Autodesk Fusion 360 part; units mm, degrees
(part 2 of 2)
  spline S177 degree 3 poles (-149.504, -22.8895) (-149.4923, -22.9168) (-149.4677, -22.974) (-149.4591, -23.0358) (-149.4546, -23.0681) knots 0 0 0 0 0.008862 0.018609 0.018609 0.018609 0.018609
  spline S178 degree 3 poles (-149.4546, -23.0681) (-149.4113, -23.0329) (-149.3307, -22.9673) (-149.2361, -22.924) (-149.1923, -22.9039) knots 0 0 0 0 0.016644 0.031058 0.031058 0.031058 0.031058
  spline S179 degree 3 poles (-149.1923, -22.9039) (-149.149, -22.8899) (-149.061, -22.8614) (-148.9686, -22.8576) (-148.9215, -22.8557) knots 0 0 0 0 0.013561 0.027613 0.027613 0.027613 0.027613
  spline S180 degree 3 poles (-148.9215, -22.8557) (-148.8489, -22.8584) (-148.7153, -22.8635) (-148.6047, -22.9378) (-148.5543, -22.9716) knots 0 0 0 0 0.021312 0.039186 0.039186 0.039186 0.039186
  spline S181 degree 3 poles (-148.5543, -22.9716) (-148.5169, -23.0135) (-148.4409, -23.0984) (-148.4307, -23.212) (-148.4255, -23.2695) knots 0 0 0 0 0.016401 0.033233 0.033233 0.033233 0.033233
  spline S182 degree 3 poles (-148.4255, -23.2695) (-148.4274, -23.3039) (-148.431, -23.3719) (-148.4595, -23.4336) (-148.4736, -23.464) knots 0 0 0 0 0.010253 0.020199 0.020199 0.020199 0.020199
  spline S183 degree 3 poles (-148.4736, -23.464) (-148.4907, -23.4917) (-148.5245, -23.5465) (-148.5752, -23.586) (-148.6002, -23.6054) knots 0 0 0 0 0.009704 0.019119 0.019119 0.019119 0.019119
  spline S184 degree 3 poles (-148.6002, -23.6054) (-148.6274, -23.6222) (-148.6829, -23.6564) (-148.7451, -23.6762) (-148.7767, -23.6862) knots 0 0 0 0 0.009559 0.019479 0.019479 0.019479 0.019479
  spline S185 degree 3 poles (-148.7767, -23.6862) (-148.8069, -23.6929) (-148.879, -23.709) (-148.9523, -23.7182) (-148.9949, -23.7235) knots 0 0 0 0 0.009264 0.022147 0.022147 0.022147 0.022147
  spline S186 degree 3 poles (-148.9949, -23.7235) (-149.0815, -23.7341) (-149.2295, -23.7523) (-149.3731, -23.7923) (-149.4327, -23.8089) knots 0 0 0 0 0.02611 0.044656 0.044656 0.044656 0.044656
  spline S187 degree 3 poles (-149.4327, -23.8089) (-149.4331, -23.8227) (-149.4336, -23.844) (-149.4338, -23.8654) (-149.4339, -23.873) knots 0 0 0 0 0.004128 0.006413 0.006413 0.006413 0.006413
  spline S188 degree 3 poles (-149.4339, -23.873) (-149.4329, -23.9174) (-149.431, -23.9956) (-149.3842, -24.0575) (-149.364, -24.0843) knots 0 0 0 0 0.012908 0.022759 0.022759 0.022759 0.022759
  spline S189 degree 3 poles (-149.364, -24.0843) (-149.326, -24.1085) (-149.2411, -24.1625) (-149.14, -24.1654) (-149.0841, -24.167) knots 0 0 0 0 0.013259 0.029661 0.029661 0.029661 0.029661
  spline S190 degree 3 poles (-149.0841, -24.167) (-149.0328, -24.1661) (-148.9427, -24.1646) (-148.8628, -24.1235) (-148.8284, -24.1058) knots 0 0 0 0 0.015134 0.026599 0.026599 0.026599 0.026599
  spline S191 degree 3 poles (-148.8284, -24.1058) (-148.8022, -24.0792) (-148.7427, -24.0187) (-148.7196, -23.9366) (-148.7068, -23.8907) knots 0 0 0 0 0.011056 0.025069 0.025069 0.025069 0.025069
  line L112 (-148.7068, -23.8907) -> (-148.4666, -23.923)
  spline S192 degree 3 poles (-148.4666, -23.923) (-148.4782, -23.9707) (-148.5, -24.0599) (-148.5504, -24.1365) (-148.5739, -24.1722) knots 0 0 0 0 0.01459 0.02731 0.02731 0.02731 0.02731
  spline S193 degree 3 poles (-148.5739, -24.1722) (-148.6029, -24.2025) (-148.6644, -24.2668) (-148.7469, -24.3007) (-148.7905, -24.3186) knots 0 0 0 0 0.012433 0.026404 0.026404 0.026404 0.026404
  spline S194 degree 3 poles (-148.7905, -24.3186) (-148.8412, -24.3336) (-148.9484, -24.3653) (-149.0602, -24.3686) (-149.1192, -24.3704) knots 0 0 0 0 0.015787 0.033398 0.033398 0.033398 0.033398
  spline S195 degree 3 poles (-149.1192, -24.3704) (-149.1757, -24.3695) (-149.2782, -24.368) (-149.3766, -24.3399) (-149.4208, -24.3273) knots 0 0 0 0 0.01685 0.030582 0.030582 0.030582 0.030582
  spline S196 degree 3 poles (-149.4208, -24.3273) (-149.4558, -24.3131) (-149.5197, -24.2873) (-149.5692, -24.2394) (-149.5915, -24.2178) knots 0 0 0 0 0.011204 0.020452 0.020452 0.020452 0.020452
  spline S197 degree 3 poles (-149.5915, -24.2178) (-149.6086, -24.1936) (-149.6443, -24.1427) (-149.66, -24.0824) (-149.6682, -24.0508) knots 0 0 0 0 0.008807 0.018509 0.018509 0.018509 0.018509
  spline S198 degree 3 poles (-149.6682, -24.0508) (-149.6718, -24.0215) (-149.6811, -23.9464) (-149.681, -23.8706) (-149.681, -23.8244) knots 0 0 0 0 0.008847 0.022698 0.022698 0.022698 0.022698
  line L113 (-149.681, -23.8244) -> (-149.6816, -23.497)
  spline S199 degree 3 poles (-149.6816, -23.497) (-149.6812, -23.4037) (-149.6806, -23.259) (-149.6935, -23.115) (-149.6981, -23.0638) knots 0 0 0 0 0.027953 0.043363 0.043363 0.043363 0.043363
  spline S200 degree 3 poles (-149.6981, -23.0638) (-149.7047, -23.0338) (-149.7181, -22.9732) (-149.7463, -22.9179) (-149.7605, -22.89) knots 0 0 0 0 0.009187 0.018535 0.018535 0.018535 0.018535
  spline S201 degree 3 poles (-144.8078, -22.2926) (-144.7279, -22.2957) (-144.5787, -22.3016) (-144.449, -22.3746) (-144.3888, -22.4085) knots 0 0 0 0 0.023612 0.044032 0.044032 0.044032 0.044032
  spline S202 degree 3 poles (-144.3888, -22.4085) (-144.3425, -22.454) (-144.2448, -22.55) (-144.2377, -22.6873) (-144.234, -22.7595) knots 0 0 0 0 0.018806 0.039631 0.039631 0.039631 0.039631
  line L114 (-144.234, -22.7595) -> (-144.4728, -22.7244)
  spline S203 degree 3 poles (-144.4728, -22.7244) (-144.4791, -22.6909) (-144.4908, -22.6286) (-144.5356, -22.5841) (-144.5563, -22.5636) knots 0 0 0 0 0.009961 0.018507 0.018507 0.018507 0.018507
  spline S204 degree 3 poles (-144.5563, -22.5636) (-144.5916, -22.5438) (-144.6689, -22.5005) (-144.7578, -22.4975) (-144.8061, -22.4959) knots 0 0 0 0 0.011961 0.026218 0.026218 0.026218 0.026218
  spline S205 degree 3 poles (-144.8061, -22.4959) (-144.8576, -22.4974) (-144.951, -22.5002) (-145.0327, -22.5447) (-145.0693, -22.5646) knots 0 0 0 0 0.015205 0.027537 0.027537 0.027537 0.027537
  spline S206 degree 3 poles (-145.0693, -22.5646) (-145.0978, -22.5902) (-145.1564, -22.6428) (-145.1815, -22.7175) (-145.1944, -22.7558) knots 0 0 0 0 0.01129 0.023203 0.023203 0.023203 0.023203
  spline S207 degree 3 poles (-145.1944, -22.7558) (-145.1997, -22.7946) (-145.2141, -22.899) (-145.2125, -23.0046) (-145.2115, -23.071) knots 0 0 0 0 0.011714 0.031602 0.031602 0.031602 0.031602
  spline S208 degree 3 poles (-145.2115, -23.071) (-145.1551, -23.0156) (-145.0434, -22.9059) (-144.8878, -22.889) (-144.8108, -22.8806) knots 0 0 0 0 0.023001 0.045538 0.045538 0.045538 0.045538
  spline S209 degree 3 poles (-144.8108, -22.8806) (-144.7177, -22.8883) (-144.5367, -22.9033) (-144.4096, -23.0325) (-144.3479, -23.0953) knots 0 0 0 0 0.027043 0.052564 0.052564 0.052564 0.052564
  spline S210 degree 3 poles (-144.3479, -23.0953) (-144.3, -23.172) (-144.2014, -23.3301) (-144.1894, -23.5162) (-144.1832, -23.612) knots 0 0 0 0 0.026695 0.054994 0.054994 0.054994 0.054994
  spline S211 degree 3 poles (-144.1832, -23.612) (-144.186, -23.6792) (-144.1913, -23.8106) (-144.2358, -23.9343) (-144.2575, -23.9948) knots 0 0 0 0 0.020023 0.0392 0.0392 0.0392 0.0392
  spline S212 degree 3 poles (-144.2575, -23.9948) (-144.2846, -24.0495) (-144.3371, -24.1559) (-144.4297, -24.23) (-144.4746, -24.2661) knots 0 0 0 0 0.018051 0.035117 0.035117 0.035117 0.035117
  spline S213 degree 3 poles (-144.4746, -24.2661) (-144.5251, -24.294) (-144.6292, -24.3516) (-144.7481, -24.3586) (-144.8094, -24.3622) knots 0 0 0 0 0.017076 0.035225 0.035225 0.035225 0.035225
  spline S214 degree 3 poles (-144.8094, -24.3622) (-144.8914, -24.3534) (-145.0572, -24.3355) (-145.1738, -24.216) (-145.2327, -24.1556) knots 0 0 0 0 0.023964 0.048437 0.048437 0.048437 0.048437
  line L115 (-145.2327, -24.1556) -> (-145.2323, -24.3303)
  line L116 (-145.2323, -24.3303) -> (-145.4588, -24.3307)
  line L117 (-145.4588, -24.3307) -> (-145.4612, -23.0783)
  spline S215 degree 3 poles (-145.4612, -23.0783) (-145.4614, -22.981) (-145.4619, -22.8174) (-145.413, -22.6617) (-145.3932, -22.5986) knots 0 0 0 0 0.028956 0.048693 0.048693 0.048693 0.048693
  spline S216 degree 3 poles (-145.3932, -22.5986) (-145.3665, -22.5537) (-145.3118, -22.4619) (-145.2215, -22.4045) (-145.1754, -22.3752) knots 0 0 0 0 0.015457 0.0316 0.0316 0.0316 0.0316
  spline S217 degree 3 poles (-145.1754, -22.3752) (-145.1206, -22.3512) (-145.0037, -22.3) (-144.8759, -22.2952) (-144.8078, -22.2926) knots 0 0 0 0 0.017756 0.037966 0.037966 0.037966 0.037966
  line L118 (-143.0208, -22.8772) -> (-142.7643, -22.8767)
  spline S218 degree 3 poles (-142.7643, -22.8767) (-142.7526, -22.904) (-142.728, -22.9612) (-142.7194, -23.023) (-142.7149, -23.0554) knots 0 0 0 0 0.008862 0.018609 0.018609 0.018609 0.018609
  spline S219 degree 3 poles (-142.7149, -23.0554) (-142.6716, -23.0201) (-142.591, -22.9545) (-142.4964, -22.9112) (-142.4526, -22.8911) knots 0 0 0 0 0.016644 0.031058 0.031058 0.031058 0.031058
  spline S220 degree 3 poles (-142.4526, -22.8911) (-142.4093, -22.8771) (-142.3213, -22.8486) (-142.2289, -22.8448) (-142.1819, -22.8429) knots 0 0 0 0 0.013561 0.027613 0.027613 0.027613 0.027613
  spline S221 degree 3 poles (-142.1819, -22.8429) (-142.1092, -22.8456) (-141.9756, -22.8507) (-141.8651, -22.925) (-141.8146, -22.9588) knots 0 0 0 0 0.021312 0.039186 0.039186 0.039186 0.039186
  spline S222 degree 3 poles (-141.8146, -22.9588) (-141.7772, -23.0007) (-141.7012, -23.0856) (-141.691, -23.1992) (-141.6858, -23.2567) knots 0 0 0 0 0.016401 0.033233 0.033233 0.033233 0.033233
  spline S223 degree 3 poles (-141.6858, -23.2567) (-141.6877, -23.2911) (-141.6913, -23.3591) (-141.7198, -23.4208) (-141.7339, -23.4512) knots 0 0 0 0 0.010253 0.020199 0.020199 0.020199 0.020199
  spline S224 degree 3 poles (-141.7339, -23.4512) (-141.751, -23.4789) (-141.7848, -23.5337) (-141.8355, -23.5732) (-141.8605, -23.5926) knots 0 0 0 0 0.009704 0.019119 0.019119 0.019119 0.019119
  spline S225 degree 3 poles (-141.8605, -23.5926) (-141.8877, -23.6094) (-141.9432, -23.6436) (-142.0054, -23.6634) (-142.037, -23.6734) knots 0 0 0 0 0.009559 0.019479 0.019479 0.019479 0.019479
  spline S226 degree 3 poles (-142.037, -23.6734) (-142.0672, -23.6801) (-142.1393, -23.6962) (-142.2126, -23.7054) (-142.2552, -23.7107) knots 0 0 0 0 0.009264 0.022147 0.022147 0.022147 0.022147
  spline S227 degree 3 poles (-142.2552, -23.7107) (-142.3418, -23.7213) (-142.4898, -23.7395) (-142.6334, -23.7795) (-142.693, -23.7961) knots 0 0 0 0 0.02611 0.044656 0.044656 0.044656 0.044656
  spline S228 degree 3 poles (-142.693, -23.7961) (-142.6934, -23.8099) (-142.6939, -23.8312) (-142.6942, -23.8526) (-142.6942, -23.8602) knots 0 0 0 0 0.004128 0.006413 0.006413 0.006413 0.006413
  spline S229 degree 3 poles (-142.6942, -23.8602) (-142.6932, -23.9046) (-142.6913, -23.9828) (-142.6445, -24.0448) (-142.6243, -24.0716) knots 0 0 0 0 0.012908 0.022759 0.022759 0.022759 0.022759
  spline S230 degree 3 poles (-142.6243, -24.0716) (-142.5863, -24.0957) (-142.5014, -24.1497) (-142.4003, -24.1526) (-142.3444, -24.1542) knots 0 0 0 0 0.013259 0.029661 0.029661 0.029661 0.029661
  spline S231 degree 3 poles (-142.3444, -24.1542) (-142.2931, -24.1533) (-142.203, -24.1518) (-142.1232, -24.1107) (-142.0888, -24.093) knots 0 0 0 0 0.015134 0.026599 0.026599 0.026599 0.026599
  spline S232 degree 3 poles (-142.0888, -24.093) (-142.0625, -24.0664) (-142.003, -24.0059) (-141.98, -23.9238) (-141.9671, -23.8779) knots 0 0 0 0 0.011056 0.025069 0.025069 0.025069 0.025069
  line L119 (-141.9671, -23.8779) -> (-141.7269, -23.9102)
  spline S233 degree 3 poles (-141.7269, -23.9102) (-141.7385, -23.9579) (-141.7603, -24.0471) (-141.8107, -24.1237) (-141.8342, -24.1594) knots 0 0 0 0 0.01459 0.02731 0.02731 0.02731 0.02731
  spline S234 degree 3 poles (-141.8342, -24.1594) (-141.8632, -24.1897) (-141.9247, -24.254) (-142.0072, -24.2879) (-142.0508, -24.3058) knots 0 0 0 0 0.012433 0.026404 0.026404 0.026404 0.026404
  spline S235 degree 3 poles (-142.0508, -24.3058) (-142.1015, -24.3208) (-142.2087, -24.3525) (-142.3206, -24.3558) (-142.3795, -24.3576) knots 0 0 0 0 0.015787 0.033398 0.033398 0.033398 0.033398
  spline S236 degree 3 poles (-142.3795, -24.3576) (-142.436, -24.3567) (-142.5385, -24.3552) (-142.6369, -24.3271) (-142.6811, -24.3145) knots 0 0 0 0 0.01685 0.030582 0.030582 0.030582 0.030582
  spline S237 degree 3 poles (-142.6811, -24.3145) (-142.7161, -24.3003) (-142.78, -24.2745) (-142.8295, -24.2266) (-142.8518, -24.205) knots 0 0 0 0 0.011204 0.020452 0.020452 0.020452 0.020452
  spline S238 degree 3 poles (-142.8518, -24.205) (-142.8689, -24.1808) (-142.9047, -24.1299) (-142.9203, -24.0696) (-142.9286, -24.038) knots 0 0 0 0 0.008807 0.018509 0.018509 0.018509 0.018509
  spline S239 degree 3 poles (-142.9286, -24.038) (-142.9322, -24.0087) (-142.9414, -23.9336) (-142.9413, -23.8578) (-142.9413, -23.8116) knots 0 0 0 0 0.008847 0.022698 0.022698 0.022698 0.022698
  line L120 (-142.9413, -23.8116) -> (-142.9419, -23.4842)
  spline S240 degree 3 poles (-142.9419, -23.4842) (-142.9415, -23.3909) (-142.9409, -23.2462) (-142.9538, -23.1022) (-142.9584, -23.051) knots 0 0 0 0 0.027953 0.043363 0.043363 0.043363 0.043363
  spline S241 degree 3 poles (-142.9584, -23.051) (-142.965, -23.021) (-142.9784, -22.9604) (-143.0066, -22.9051) (-143.0208, -22.8772) knots 0 0 0 0 0.009187 0.018535 0.018535 0.018535 0.018535
  spline S242 degree 3 poles (-148.8692, -25.9756) (-148.7958, -25.9798) (-148.6557, -25.9878) (-148.5405, -26.0673) (-148.4856, -26.1052) knots 0 0 0 0 0.021564 0.041189 0.041189 0.041189 0.041189
  spline S243 degree 3 poles (-148.4856, -26.1052) (-148.4407, -26.1548) (-148.346, -26.2593) (-148.3199, -26.3982) (-148.3062, -26.4712) knots 0 0 0 0 0.01968 0.041471 0.041471 0.041471 0.041471
  line L121 (-148.3062, -26.4712) -> (-148.5421, -26.4934)
  spline S244 degree 3 poles (-148.5421, -26.4934) (-148.5527, -26.4436) (-148.5717, -26.3535) (-148.6308, -26.2834) (-148.6572, -26.2522) knots 0 0 0 0 0.015008 0.027097 0.027097 0.027097 0.027097
  spline S245 degree 3 poles (-148.6572, -26.2522) (-148.6883, -26.2304) (-148.7533, -26.1848) (-148.8328, -26.18) (-148.8743, -26.1776) knots 0 0 0 0 0.011173 0.023358 0.023358 0.023358 0.023358
  spline S246 degree 3 poles (-148.8743, -26.1776) (-148.9103, -26.1795) (-148.9801, -26.1832) (-149.0425, -26.2146) (-149.0727, -26.2298) knots 0 0 0 0 0.010703 0.020715 0.020715 0.020715 0.020715
  spline S247 degree 3 poles (-149.0727, -26.2298) (-149.0998, -26.2487) (-149.1545, -26.2867) (-149.1929, -26.3411) (-149.2122, -26.3685) knots 0 0 0 0 0.009841 0.019815 0.019815 0.019815 0.019815
  spline S248 degree 3 poles (-149.2122, -26.3685) (-149.2301, -26.402) (-149.2698, -26.4763) (-149.2913, -26.5579) (-149.3032, -26.6027) knots 0 0 0 0 0.011348 0.025194 0.025194 0.025194 0.025194
  spline S249 degree 3 poles (-149.3032, -26.6027) (-149.3138, -26.6521) (-149.3352, -26.751) (-149.338, -26.8522) (-149.3394, -26.9029) knots 0 0 0 0 0.015125 0.030296 0.030296 0.030296 0.030296
  spline S250 degree 3 poles (-149.3394, -26.9029) (-149.3394, -26.9097) (-149.3391, -26.9261) (-149.3384, -26.9424) (-149.338, -26.952) knots 0 0 0 0 0.002047 0.004913 0.004913 0.004913 0.004913
  spline S251 degree 3 poles (-149.338, -26.952) (-149.3109, -26.9145) (-149.256, -26.8383) (-149.1772, -26.7872) (-149.1371, -26.7613) knots 0 0 0 0 0.013741 0.027912 0.027912 0.027912 0.027912
  spline S252 degree 3 poles (-149.1371, -26.7613) (-149.0937, -26.7399) (-149.0065, -26.697) (-148.9096, -26.6909) (-148.861, -26.6878) knots 0 0 0 0 0.014368 0.028825 0.028825 0.028825 0.028825
  spline S253 degree 3 poles (-148.861, -26.6878) (-148.7814, -26.6951) (-148.622, -26.7099) (-148.501, -26.8146) (-148.4405, -26.867) knots 0 0 0 0 0.023358 0.04675 0.04675 0.04675 0.04675
  spline S254 degree 3 poles (-148.4405, -26.867) (-148.3902, -26.9339) (-148.2848, -27.0741) (-148.2736, -27.2496) (-148.2677, -27.3415) knots 0 0 0 0 0.024534 0.051481 0.051481 0.051481 0.051481
  spline S255 degree 3 poles (-148.2677, -27.3415) (-148.2735, -27.4364) (-148.2846, -27.6179) (-148.394, -27.7626) (-148.4461, -27.8316) knots 0 0 0 0 0.02782 0.053201 0.053201 0.053201 0.053201
  spline S256 degree 3 poles (-148.4461, -27.8316) (-148.5102, -27.8858) (-148.6399, -27.9957) (-148.8095, -28.0105) (-148.8953, -28.018) knots 0 0 0 0 0.024536 0.049711 0.049711 0.049711 0.049711
  spline S257 degree 3 poles (-148.8953, -28.018) (-148.9589, -28.0138) (-149.0856, -28.0054) (-149.1968, -27.9441) (-149.2523, -27.9136) knots 0 0 0 0 0.018857 0.037596 0.037596 0.037596 0.037596
  spline S258 degree 3 poles (-149.2523, -27.9136) (-149.3033, -27.8742) (-149.408, -27.7933) (-149.4678, -27.6752) (-149.4984, -27.6146) knots 0 0 0 0 0.019093 0.039165 0.039165 0.039165 0.039165
  spline S259 degree 3 poles (-149.4984, -27.6146) (-149.5229, -27.5359) (-149.5798, -27.3531) (-149.5821, -27.1613) (-149.5834, -27.052) knots 0 0 0 0 0.024607 0.057161 0.057161 0.057161 0.057161
  spline S260 degree 3 poles (-149.5834, -27.052) (-149.582, -26.9365) (-149.5797, -26.7293) (-149.5253, -26.5297) (-149.5013, -26.4414) knots 0 0 0 0 0.034493 0.061835 0.061835 0.061835 0.061835
  spline S261 degree 3 poles (-149.5013, -26.4414) (-149.4717, -26.3712) (-149.4152, -26.237) (-149.3063, -26.1409) (-149.2544, -26.0951) knots 0 0 0 0 0.022523 0.043023 0.043023 0.043023 0.043023
  spline S262 degree 3 poles (-149.2544, -26.0951) (-149.1964, -26.0603) (-149.0779, -25.9892) (-148.9398, -25.9802) (-148.8692, -25.9756) knots 0 0 0 0 0.019951 0.040848 0.040848 0.040848 0.040848
  spline S263 degree 3 poles (-146.7002, -26.5841) (-146.7034, -26.6454) (-146.7095, -26.7626) (-146.7697, -26.863) (-146.7984, -26.911) knots 0 0 0 0 0.018093 0.034604 0.034604 0.034604 0.034604
  spline S264 degree 3 poles (-146.7984, -26.911) (-146.8359, -26.9517) (-146.9137, -27.0363) (-147.0231, -27.0723) (-147.0798, -27.0909) knots 0 0 0 0 0.016316 0.033898 0.033898 0.033898 0.033898
  spline S265 degree 3 poles (-147.0798, -27.0909) (-147.0331, -27.1102) (-146.9454, -27.1464) (-146.8825, -27.2171) (-146.8531, -27.2501) knots 0 0 0 0 0.014933 0.028029 0.028029 0.028029 0.028029
  spline S266 degree 3 poles (-146.8531, -27.2501) (-146.8315, -27.2871) (-146.7869, -27.3638) (-146.7816, -27.4524) (-146.7789, -27.4983) knots 0 0 0 0 0.012661 0.026224 0.026224 0.026224 0.026224
  spline S267 degree 3 poles (-146.7789, -27.4983) (-146.7852, -27.5681) (-146.7979, -27.7073) (-146.8894, -27.8129) (-146.9351, -27.8656) knots 0 0 0 0 0.020468 0.040823 0.040823 0.040823 0.040823
  spline S268 degree 3 poles (-146.9351, -27.8656) (-146.9937, -27.909) (-147.1173, -28.0007) (-147.2713, -28.0101) (-147.3523, -28.0151) knots 0 0 0 0 0.021415 0.045172 0.045172 0.045172 0.045172
  spline S269 degree 3 poles (-147.3523, -28.0151) (-147.4339, -28.0102) (-147.5897, -28.0009) (-147.7147, -27.908) (-147.7741, -27.8637) knots 0 0 0 0 0.02394 0.045691 0.045691 0.045691 0.045691
  spline S270 degree 3 poles (-147.7741, -27.8637) (-147.8208, -27.8105) (-147.9138, -27.7042) (-147.9276, -27.5637) (-147.9345, -27.4936) knots 0 0 0 0 0.020682 0.041247 0.041247 0.041247 0.041247
  spline S271 degree 3 poles (-147.9345, -27.4936) (-147.9318, -27.4492) (-147.9267, -27.3627) (-147.8831, -27.2878) (-147.8619, -27.2514) knots 0 0 0 0 0.013139 0.025609 0.025609 0.025609 0.025609
  spline S272 degree 3 poles (-147.8619, -27.2514) (-147.8331, -27.2184) (-147.7718, -27.1483) (-147.686, -27.1115) (-147.6405, -27.092) knots 0 0 0 0 0.012951 0.027588 0.027588 0.027588 0.027588
  spline S273 degree 3 poles (-147.6405, -27.092) (-147.6975, -27.0701) (-147.8067, -27.0281) (-147.8842, -26.9406) (-147.9213, -26.8988) knots 0 0 0 0 0.018015 0.034524 0.034524 0.034524 0.034524
  spline S274 degree 3 poles (-147.9213, -26.8988) (-147.9494, -26.8512) (-148.0075, -26.7528) (-148.0145, -26.6387) (-148.018, -26.5798) knots 0 0 0 0 0.016344 0.033768 0.033768 0.033768 0.033768
  spline S275 degree 3 poles (-148.018, -26.5798) (-148.0108, -26.4978) (-147.9964, -26.3348) (-147.8902, -26.2102) (-147.8374, -26.1483) knots 0 0 0 0 0.024034 0.04782 0.04782 0.04782 0.04782
  spline S276 degree 3 poles (-147.8374, -26.1483) (-147.7702, -26.0973) (-147.6294, -25.9904) (-147.4526, -25.9788) (-147.3603, -25.9728) knots 0 0 0 0 0.024757 0.051851 0.051851 0.051851 0.051851
  spline S277 degree 3 poles (-147.3603, -25.9728) (-147.2678, -25.9785) (-147.0909, -25.9895) (-146.9498, -26.0962) (-146.8824, -26.1472) knots 0 0 0 0 0.027096 0.051881 0.051881 0.051881 0.051881
  spline S278 degree 3 poles (-146.8824, -26.1472) (-146.8294, -26.2096) (-146.7222, -26.3357) (-146.7076, -26.5007) (-146.7002, -26.5841) knots 0 0 0 0 0.02394 0.048393 0.048393 0.048393 0.048393
  spline S279 degree 3 poles (-144.2237, -25.9668) (-144.1332, -25.9744) (-143.9567, -25.9891) (-143.8305, -26.113) (-143.769, -26.1733) knots 0 0 0 0 0.026334 0.051363 0.051363 0.051363 0.051363
  spline S280 degree 3 poles (-143.769, -26.1733) (-143.7115, -26.2804) (-143.5759, -26.5326) (-143.572, -26.8205) (-143.5697, -26.986) knots 0 0 0 0 0.036009 0.08476 0.08476 0.08476 0.08476
  spline S281 degree 3 poles (-143.5697, -26.986) (-143.5709, -27.0934) (-143.5732, -27.2867) (-143.6205, -27.4739) (-143.6416, -27.5571) knots 0 0 0 0 0.032061 0.057736 0.057736 0.057736 0.057736
  spline S282 degree 3 poles (-143.6416, -27.5571) (-143.6673, -27.6239) (-143.7161, -27.7506) (-143.8124, -27.846) (-143.8579, -27.8911) knots 0 0 0 0 0.021191 0.040192 0.040192 0.040192 0.040192
  spline S283 degree 3 poles (-143.8579, -27.8911) (-143.9104, -27.9254) (-144.0202, -27.9972) (-144.1514, -28.005) (-144.2199, -28.0091) knots 0 0 0 0 0.018481 0.038665 0.038665 0.038665 0.038665
  spline S284 degree 3 poles (-144.2199, -28.0091) (-144.271, -28.007) (-144.3692, -28.0029) (-144.4592, -27.9636) (-144.5024, -27.9448) knots 0 0 0 0 0.015196 0.029197 0.029197 0.029197 0.029197
  spline S285 degree 3 poles (-144.5024, -27.9448) (-144.5413, -27.9206) (-144.6204, -27.8715) (-144.6754, -27.7964) (-144.7033, -27.7583) knots 0 0 0 0 0.013619 0.027641 0.027641 0.027641 0.027641
  spline S286 degree 3 poles (-144.7033, -27.7583) (-144.7287, -27.714) (-144.7825, -27.6201) (-144.8123, -27.5161) (-144.828, -27.4611) knots 0 0 0 0 0.01527 0.032333 0.032333 0.032333 0.032333
  spline S287 degree 3 poles (-144.828, -27.4611) (-144.8412, -27.3927) (-144.8713, -27.2368) (-144.873, -27.0778) (-144.8739, -26.9885) knots 0 0 0 0 0.020858 0.04757 0.04757 0.04757 0.04757
  spline S288 degree 3 poles (-144.8739, -26.9885) (-144.8726, -26.8819) (-144.8704, -26.6896) (-144.8235, -26.5032) (-144.8027, -26.4202) knots 0 0 0 0 0.031856 0.057454 0.057454 0.057454 0.057454
  spline S289 degree 3 poles (-144.8027, -26.4202) (-144.7771, -26.3533) (-144.7286, -26.2265) (-144.6325, -26.1308) (-144.5871, -26.0855) knots 0 0 0 0 0.021185 0.040213 0.040213 0.040213 0.040213
  spline S290 degree 3 poles (-144.5871, -26.0855) (-144.5345, -26.051) (-144.4243, -25.9788) (-144.2926, -25.9709) (-144.2237, -25.9668) knots 0 0 0 0 0.018535 0.038823 0.038823 0.038823 0.038823
  spline S291 degree 3 poles (-140.9528, -26.3317) (-140.9886, -26.3949) (-141.0772, -26.5513) (-141.0764, -26.7327) (-141.076, -26.8408) knots 0 0 0 0 0.021463 0.053164 0.053164 0.053164 0.053164
  line L122 (-141.076, -26.8408) -> (-141.0738, -27.9949)
  line L123 (-141.0738, -27.9949) -> (-141.3385, -27.9954)
  line L124 (-141.3385, -27.9954) -> (-141.3406, -26.8399)
  spline S292 degree 3 poles (-141.3406, -26.8399) (-141.3396, -26.7491) (-141.3376, -26.5863) (-141.293, -26.43) (-141.2733, -26.3609) knots 0 0 0 0 0.0271 0.048558 0.048558 0.048558 0.048558
  spline S293 degree 3 poles (-141.2733, -26.3609) (-141.2454, -26.3041) (-141.1879, -26.1872) (-141.082, -26.111) (-141.0276, -26.0719) knots 0 0 0 0 0.018712 0.038457 0.038457 0.038457 0.038457
  spline S294 degree 3 poles (-141.0276, -26.0719) (-140.9602, -26.0394) (-140.813, -25.9685) (-140.6493, -25.9629) (-140.5606, -25.9599) knots 0 0 0 0 0.022208 0.048498 0.048498 0.048498 0.048498
  spline S295 degree 3 poles (-140.5606, -25.9599) (-140.4742, -25.9622) (-140.3148, -25.9665) (-140.1679, -26.0278) (-140.1007, -26.0558) knots 0 0 0 0 0.02566 0.047343 0.047343 0.047343 0.047343
  spline S296 degree 3 poles (-140.1007, -26.0558) (-140.0454, -26.0915) (-139.9354, -26.1622) (-139.875, -26.2781) (-139.845, -26.3357) knots 0 0 0 0 0.019364 0.038493 0.038493 0.038493 0.038493
  spline S297 degree 3 poles (-139.845, -26.3357) (-139.8227, -26.4075) (-139.772, -26.5705) (-139.7692, -26.7414) (-139.7677, -26.8369) knots 0 0 0 0 0.022452 0.050944 0.050944 0.050944 0.050944
  line L125 (-139.7677, -26.8369) -> (-139.7655, -27.9925)
  line L126 (-139.7655, -27.9925) -> (-140.0301, -27.993)
  line L127 (-140.0301, -27.993) -> (-140.0323, -26.8388)
  spline S298 degree 3 poles (-140.0323, -26.8388) (-140.0327, -26.7628) (-140.0334, -26.6326) (-140.0674, -26.5071) (-140.0815, -26.4549) knots 0 0 0 0 0.022662 0.038849 0.038849 0.038849 0.038849
  spline S299 degree 3 poles (-140.0815, -26.4549) (-140.1007, -26.416) (-140.1394, -26.3379) (-140.2119, -26.2893) (-140.2483, -26.2649) knots 0 0 0 0 0.01276 0.025677 0.025677 0.025677 0.025677
  spline S300 degree 3 poles (-140.2483, -26.2649) (-140.2914, -26.2455) (-140.383, -26.2042) (-140.4836, -26.2005) (-140.537, -26.1986) knots 0 0 0 0 0.01404 0.029868 0.029868 0.029868 0.029868
  spline S301 degree 3 poles (-140.537, -26.1986) (-140.6234, -26.2007) (-140.7763, -26.2044) (-140.8994, -26.2932) (-140.9528, -26.3317) knots 0 0 0 0 0.025218 0.044567 0.044567 0.044567 0.044567
  spline S302 degree 3 poles (-153.5723, -29.3325) (-153.6428, -29.3373) (-153.78, -29.3467) (-153.8935, -29.4239) (-153.9486, -29.4614) knots 0 0 0 0 0.020781 0.040419 0.040419 0.040419 0.040419
  spline S303 degree 3 poles (-153.9486, -29.4614) (-153.9963, -29.512) (-154.0985, -29.6205) (-154.1364, -29.7652) (-154.1566, -29.8424) knots 0 0 0 0 0.020513 0.044031 0.044031 0.044031 0.044031
  line L128 (-154.1566, -29.8424) -> (-154.4214, -29.7761)
  spline S304 degree 3 poles (-154.4214, -29.7761) (-154.3905, -29.6755) (-154.3317, -29.4847) (-154.19, -29.3446) (-154.1229, -29.2783) knots 0 0 0 0 0.031005 0.058853 0.058853 0.058853 0.058853
  spline S305 degree 3 poles (-154.1229, -29.2783) (-154.0453, -29.2282) (-153.8845, -29.1245) (-153.6934, -29.1123) (-153.5946, -29.106) knots 0 0 0 0 0.027244 0.056397 0.056397 0.056397 0.056397
  spline S306 degree 3 poles (-153.5946, -29.106) (-153.4949, -29.1094) (-153.3099, -29.1157) (-153.1447, -29.1985) (-153.0684, -29.2367) knots 0 0 0 0 0.029499 0.054784 0.054784 0.054784 0.054784
  spline S307 degree 3 poles (-153.0684, -29.2367) (-153.0043, -29.2866) (-152.8721, -29.3895) (-152.7977, -29.5399) (-152.7594, -29.6174) knots 0 0 0 0 0.024039 0.049604 0.049604 0.049604 0.049604
  spline S308 degree 3 poles (-152.7594, -29.6174) (-152.7284, -29.7028) (-152.6655, -29.8759) (-152.657, -30.06) (-152.6526, -30.1534) knots 0 0 0 0 0.027074 0.054928 0.054928 0.054928 0.054928
  spline S309 degree 3 poles (-152.6526, -30.1534) (-152.6564, -30.2522) (-152.6637, -30.4411) (-152.7363, -30.6155) (-152.771, -30.6986) knots 0 0 0 0 0.029398 0.056194 0.056194 0.056194 0.056194
  spline S310 degree 3 poles (-152.771, -30.6986) (-152.8144, -30.7713) (-152.9004, -30.9153) (-153.0406, -31.0071) (-153.11, -31.0526) knots 0 0 0 0 0.025058 0.049588 0.049588 0.049588 0.049588
  spline S311 degree 3 poles (-153.11, -31.0526) (-153.1858, -31.0879) (-153.3395, -31.1596) (-153.5089, -31.1693) (-153.5948, -31.1742) knots 0 0 0 0 0.02485 0.050387 0.050387 0.050387 0.050387
  spline S312 degree 3 poles (-153.5948, -31.1742) (-153.6892, -31.1692) (-153.8702, -31.1597) (-154.0255, -31.0668) (-154.0998, -31.0224) knots 0 0 0 0 0.027889 0.053453 0.053453 0.053453 0.053453
  spline S313 degree 3 poles (-154.0998, -31.0224) (-154.1634, -30.965) (-154.2948, -30.8463) (-154.3548, -30.6794) (-154.3858, -30.5932) knots 0 0 0 0 0.025285 0.052286 0.052286 0.052286 0.052286
  line L129 (-154.3858, -30.5932) -> (-154.1253, -30.5313)
  spline S314 degree 3 poles (-154.1253, -30.5313) (-154.1016, -30.5973) (-154.0579, -30.7188) (-153.9652, -30.808) (-153.9228, -30.8488) knots 0 0 0 0 0.020699 0.03811 0.03811 0.03811 0.03811
  spline S315 degree 3 poles (-153.9228, -30.8488) (-153.8742, -30.8777) (-153.7718, -30.9388) (-153.6525, -30.9447) (-153.5897, -30.9478) knots 0 0 0 0 0.016702 0.035219 0.035219 0.035219 0.035219
  spline S316 degree 3 poles (-153.5897, -30.9478) (-153.5175, -30.9441) (-153.3802, -30.937) (-153.261, -30.8689) (-153.2045, -30.8365) knots 0 0 0 0 0.021343 0.040595 0.040595 0.040595 0.040595
  spline S317 degree 3 poles (-153.2045, -30.8365) (-153.1567, -30.7962) (-153.0603, -30.7148) (-153.0119, -30.5982) (-152.9875, -30.5394) knots 0 0 0 0 0.018474 0.037274 0.037274 0.037274 0.037274
  spline S318 degree 3 poles (-152.9875, -30.5394) (-152.9693, -30.4768) (-152.9329, -30.3512) (-152.9279, -30.2207) (-152.9255, -30.1552) knots 0 0 0 0 0.019489 0.039044 0.039044 0.039044 0.039044
  spline S319 degree 3 poles (-152.9255, -30.1552) (-152.928, -30.0749) (-152.9327, -29.923) (-152.9789, -29.7782) (-153.0007, -29.71) knots 0 0 0 0 0.023964 0.045355 0.045355 0.045355 0.045355
  spline S320 degree 3 poles (-153.0007, -29.71) (-153.0282, -29.6511) (-153.0816, -29.5368) (-153.1832, -29.4621) (-153.2325, -29.4259) knots 0 0 0 0 0.019149 0.037185 0.037185 0.037185 0.037185
  spline S321 degree 3 poles (-153.2325, -29.4259) (-153.2859, -29.3986) (-153.3927, -29.3439) (-153.5125, -29.3363) (-153.5723, -29.3325) knots 0 0 0 0 0.017797 0.035586 0.035586 0.035586 0.035586
  line L130 (-150.3225, -29.3699) -> (-150.3229, -29.1339)
  line L131 (-150.3229, -29.1339) -> (-148.8304, -29.1311)
  line L132 (-148.8304, -29.1311) -> (-148.8266, -31.1311)
  line L133 (-148.8266, -31.1311) -> (-150.2728, -31.1338)
  line L134 (-150.2728, -31.1338) -> (-150.2732, -30.8978)
  line L135 (-150.2732, -30.8978) -> (-149.0918, -30.8956)
  line L136 (-149.0918, -30.8956) -> (-149.0929, -30.283)
  line L137 (-149.0929, -30.283) -> (-150.1993, -30.2851)
  line L138 (-150.1993, -30.2851) -> (-150.1998, -30.0505)
  line L139 (-150.1998, -30.0505) -> (-149.0934, -30.0484)
  line L140 (-149.0934, -30.0484) -> (-149.0947, -29.3676)
  line L141 (-149.0947, -29.3676) -> (-150.3225, -29.3699)
  line L142 (-146.0002, -30.8897) -> (-146.0036, -29.1257)
  line L143 (-146.0036, -29.1257) -> (-145.7389, -29.1252)
  line L144 (-145.7389, -29.1252) -> (-145.7356, -30.8892)
  line L145 (-145.7356, -30.8892) -> (-145.0766, -30.888)
  line L146 (-145.0766, -30.888) -> (-145.0762, -31.124)
  line L147 (-145.0762, -31.124) -> (-146.6615, -31.127)
  line L148 (-146.6615, -31.127) -> (-146.6619, -30.891)
  line L149 (-146.6619, -30.891) -> (-146.0002, -30.8897)
  line L150 (-142.9758, -29.356) -> (-142.9762, -29.12)
  line L151 (-142.9762, -29.12) -> (-141.4837, -29.1171)
  line L152 (-141.4837, -29.1171) -> (-141.4799, -31.1171)
  line L153 (-141.4799, -31.1171) -> (-142.926, -31.1199)
  line L154 (-142.926, -31.1199) -> (-142.9265, -30.8839)
  line L155 (-142.9265, -30.8839) -> (-141.745, -30.8816)
  line L156 (-141.745, -30.8816) -> (-141.7462, -30.2691)
  line L157 (-141.7462, -30.2691) -> (-142.8526, -30.2712)
  line L158 (-142.8526, -30.2712) -> (-142.8531, -30.0365)
  line L159 (-142.8531, -30.0365) -> (-141.7466, -30.0344)
  line L160 (-141.7466, -30.0344) -> (-141.7479, -29.3537)
  line L161 (-141.7479, -29.3537) -> (-142.9758, -29.356)
  line L162 (-160, -62.5) -> (-147, -62.5)
  line L163 (-147, -62.5) -> (-147, -59.5)
  line L164 (-147, -59.5) -> (-103.5, -59.5)
  line L165 (-103.5, -59.5) -> (-103.5, -77.5)
  line L166 (-103.5, -77.5) -> (-147, -77.5)
  line L167 (-147, -77.5) -> (-147, -74.5)
  line L168 (-147, -74.5) -> (-160, -74.5)
  line L169 (-160, -74.5) -> (-160, -80)
  line L170 (-160, -80) -> (0, -80)
  line L171 (0, -80) -> (0, -68.487)
  line L172 (0, -68.487) -> (-1.5, -68.487)
  line L173 (-1.5, -68.487) -> (-1.5, -72.487)
  line L174 (-1.5, -72.487) -> (-19.5, -72.487)
  line L175 (-19.5, -72.487) -> (-19.5, -54.487)
  line L176 (-19.5, -54.487) -> (-1.5, -54.487)
  line L177 (-1.5, -54.487) -> (-1.5, -58.487)
  line L178 (-1.5, -58.487) -> (0, -58.487)
  line L179 (0, -58.487) -> (0, 0)
  line L180 (0, 0) -> (-144, 0)
  line L181 (-144, 0) -> (-144, -2)
  line L182 (-144, -2) -> (-140, -2)
  line L183 (-140, -2) -> (-140, -20)
  line L184 (-140, -20) -> (-158, -20)
  line L185 (-158, -20) -> (-158, -2)
  line L186 (-158, -2) -> (-154, -2)
  line L187 (-154, -2) -> (-154, 0)
  line L188 (-154, 0) -> (-160, 0)
  line L189 (-160, 0) -> (-160, -38)
  line L190 (-160, -38) -> (-157.5, -38)
  line L191 (-157.5, -38) -> (-157.5, -34)
  line L192 (-157.5, -34) -> (-139.5, -34)
  line L193 (-139.5, -34) -> (-139.5, -52)
  line L194 (-139.5, -52) -> (-157.5, -52)
  line L195 (-157.5, -52) -> (-157.5, -48)
  line L196 (-157.5, -48) -> (-160, -48)
  line L197 (-160, -48) -> (-160, -62.5)
  line L198 (-22, -52) -> (-27.5, -52)
  line L199 (-27.5, -52) -> (-27.5, -46.5)
  line L200 (-27.5, -46.5) -> (-22, -46.5)
  line L201 (-22, -46.5) -> (-22, -52)
  line L202 (-22, -1.5) -> (-60.5, -1.5)
  line L203 (-60.5, -1.5) -> (-60.5, -52)
  line L204 (-60.5, -52) -> (-22, -52)
  line L205 (-22, -52) -> (-22, -1.5)
  line L206 (-60.5, -52) -> (-55, -52)
  line L207 (-55, -52) -> (-55, -46.5)
  line L208 (-55, -46.5) -> (-60.5, -46.5)
  line L209 (-60.5, -46.5) -> (-60.5, -52)
  line L210 (-22, -1.5) -> (-27.5, -1.5)
  line L211 (-27.5, -1.5) -> (-27.5, -7)
  line L212 (-27.5, -7) -> (-22, -7)
  line L213 (-22, -7) -> (-22, -1.5)
  line L214 (-60.5, -1.5) -> (-55, -1.5)
  line L215 (-55, -1.5) -> (-55, -7)
  line L216 (-55, -7) -> (-60.5, -7)
  line L217 (-60.5, -7) -> (-60.5, -1.5)
  line L218 (-62.5, -52) -> (-68, -52)
  line L219 (-68, -52) -> (-68, -46.5)
  line L220 (-68, -46.5) -> (-62.5, -46.5)
  line L221 (-62.5, -46.5) -> (-62.5, -52)
  line L222 (-62.5, -1.5) -> (-68, -1.5)
  line L223 (-68, -1.5) -> (-68, -7)
  line L224 (-68, -7) -> (-62.5, -7)
  line L225 (-62.5, -7) -> (-62.5, -1.5)
  line L226 (-137.5, -52) -> (-132, -52)
  line L227 (-132, -52) -> (-132, -46.5)
  line L228 (-132, -46.5) -> (-137.5, -46.5)
  line L229 (-137.5, -46.5) -> (-137.5, -52)
  line L230 (-137.5, -1.5) -> (-132, -1.5)
  line L231 (-132, -1.5) -> (-132, -7)
  line L232 (-132, -7) -> (-137.5, -7)
  line L233 (-137.5, -7) -> (-137.5, -1.5)
  line L234 (-75, -77.5) -> (-80.5, -77.5)
  line L235 (-80.5, -77.5) -> (-80.5, -72)
  line L236 (-80.5, -72) -> (-75, -72)
  line L237 (-75, -72) -> (-75, -77.5)
  line L238 (-75, -55.2) -> (-80.5, -55.2)
  line L239 (-80.5, -55.2) -> (-80.5, -60.7)
  line L240 (-80.5, -60.7) -> (-75, -60.7)
  line L241 (-75, -60.7) -> (-75, -55.2)
  line L242 (-100.5, -77.5) -> (-95, -77.5)
  line L243 (-95, -77.5) -> (-95, -72)
  line L244 (-95, -72) -> (-100.5, -72)
  line L245 (-100.5, -72) -> (-100.5, -77.5)
  line L246 (-100.5, -55.2) -> (-95, -55.2)
  line L247 (-95, -55.2) -> (-95, -60.7)
  line L248 (-95, -60.7) -> (-100.5, -60.7)
  line L249 (-100.5, -60.7) -> (-100.5, -55.2)
  line L250 (-157.5, -52) -> (-153.8, -52)
  line L251 (-153.8, -52) -> (-153.8, -48.3)
  line L252 (-153.8, -48.3) -> (-157.5, -48.3)
  line L253 (-157.5, -48.3) -> (-157.5, -52)
  line L254 (-157.5, -34) -> (-153.8, -34)
  line L255 (-153.8, -34) -> (-153.8, -37.7)
  line L256 (-153.8, -37.7) -> (-157.5, -37.7)
  line L257 (-157.5, -37.7) -> (-157.5, -34)
  line L258 (-140, -2) -> (-143.7, -2)
  line L259 (-143.7, -2) -> (-143.7, -5.7)
  line L260 (-143.7, -5.7) -> (-140, -5.7)
  line L261 (-140, -5.7) -> (-140, -2)
  line L262 (-158, -2) -> (-154.3, -2)
  line L263 (-154.3, -2) -> (-154.3, -5.7)
  line L264 (-154.3, -5.7) -> (-158, -5.7)
  line L265 (-158, -5.7) -> (-158, -2)
  line L266 (-1.5, -72.487) -> (-5.2, -72.487)
  line L267 (-5.2, -72.487) -> (-5.2, -68.787)
  line L268 (-5.2, -68.787) -> (-1.5, -68.787)
  line L269 (-1.5, -68.787) -> (-1.5, -72.487)
  line L270 (-1.5, -54.487) -> (-5.2, -54.487)
  line L271 (-5.2, -54.487) -> (-5.2, -58.187)
  line L272 (-5.2, -58.187) -> (-1.5, -58.187)
  line L273 (-1.5, -58.187) -> (-1.5, -54.487)
  line L274 (-103.5, -77.5) -> (-106, -77.5)
  line L275 (-106, -77.5) -> (-106, -75)
  line L276 (-106, -75) -> (-103.5, -75)
  line L277 (-103.5, -75) -> (-103.5, -77.5)
  line L278 (-103.5, -59.5) -> (-106, -59.5)
  line L279 (-106, -59.5) -> (-106, -62)
  line L280 (-106, -62) -> (-103.5, -62)
  line L281 (-103.5, -62) -> (-103.5, -59.5)
  line L282 (-147, -77.5) -> (-144.5, -77.5)
  line L283 (-144.5, -77.5) -> (-144.5, -75)
  line L284 (-144.5, -75) -> (-147, -75)
  line L285 (-147, -75) -> (-147, -77.5)
  line L286 (-147, -59.5) -> (-144.5, -59.5)
  line L287 (-144.5, -59.5) -> (-144.5, -62)
  line L288 (-144.5, -62) -> (-147, -62)
  line L289 (-147, -62) -> (-147, -59.5)
  circle A4 centre (-24.75, -49.25) radius 1.5
  circle A5 centre (-3.35, -70.637) radius 1
  circle A6 centre (-3.35, -56.337) radius 1
  circle A7 centre (-57.75, -49.25) radius 1.5
  circle A8 centre (-57.75, -4.25) radius 1.5
  circle A9 centre (-24.75, -4.25) radius 1.5
  circle A10 centre (-65.25, -49.25) radius 1.5
  circle A11 centre (-134.75, -49.25) radius 1.5
  circle A12 centre (-134.75, -4.25) radius 1.5
  circle A13 centre (-65.25, -4.25) radius 1.5
  circle A14 centre (-141.85, -3.85) radius 1
  circle A15 centre (-156.15, -3.85) radius 1
  circle A16 centre (-155.65, -50.15) radius 1
  circle A17 centre (-155.65, -35.85) radius 1
  circle A18 centre (-77.75, -74.75) radius 1
  circle A19 centre (-77.75, -57.95) radius 1
  circle A20 centre (-97.75, -74.75) radius 1
  circle A21 centre (-97.75, -57.95) radius 1
  circle A22 centre (-104.75, -76.25) radius 0.75
  circle A23 centre (-145.75, -76.25) radius 0.75
  circle A24 centre (-145.75, -60.75) radius 0.75
  circle A25 centre (-104.75, -60.75) radius 0.75
  dimension "d196" = 5.5
  dimension "d197" = 5.5
  dimension "d198" = 5.5
  dimension "d199" = 5.5
  dimension "d200" = 5.5
  dimension "d201" = 5.5
  dimension "d202" = 5.5
  dimension "d203" = 5.5
  dimension "d204" = 5.5
  dimension "d205" = 5.5
  dimension "d206" = 5.5
  dimension "d207" = 5.5
  dimension "d208" = 5.5
  dimension "d209" = 5.5
  dimension "d210" = 5.5
  dimension "d211" = 5.5
  dimension "d212" = 5.5
  dimension "d213" = 5.5
  dimension "d214" = 5.5
  dimension "d215" = 5.5
  dimension "d216" = 5.5
  dimension "d217" = 5.5
  dimension "d218" = 5.5
  dimension "d219" = 5.5
  dimension "d220" = 3.7
  dimension "d221" = 3.7
  dimension "d222" = 3.7
  dimension "d223" = 3.7
  dimension "d224" = 3.7
  dimension "d225" = 3.7
  dimension "d226" = 3.7
  dimension "d227" = 3.7
  dimension "d228" = 3.7
  dimension "d229" = 3.7
  dimension "d230" = 3.7
  dimension "d231" = 3.7
  dimension "d232" = 2.5
  dimension "d233" = 2.5
  dimension "d234" = 2.5
  dimension "d235" = 2.5
  dimension "d236" = 2.5
  dimension "d237" = 2.5
  dimension "d238" = 2.5
  dimension "d239" = 2.5
  dimension "d240" = 3
  dimension "d243" = 2
  dimension "d244" = 2
  dimension "d245" = 3
  dimension "d246" = 3
  dimension "d247" = 3
  dimension "d248" = 3
  dimension "d249" = 3
  dimension "d250" = 3
  dimension "d251" = 3
  dimension "d252" = 2
  dimension "d253" = 2
  dimension "d254" = 2
  dimension "d255" = 2
  dimension "d256" = 2
  dimension "d257" = 2
  dimension "d258" = 2
  dimension "d259" = 2
  dimension "d260" = 1.5
  dimension "d261" = 1.5
  dimension "d262" = 1.5
  dimension "d263" = 1.5
  constraint horizontal L198
  constraint vertical L199
  constraint horizontal L200
  constraint vertical L201
  constraint coincident L92.end L93.start
  constraint horizontal L206
  constraint vertical L207
  constraint horizontal L208
  constraint vertical L209
  constraint coincident L90.start L93.end
  constraint horizontal L210
  constraint vertical L211
  constraint horizontal L212
  constraint vertical L213
  constraint coincident L91.end L92.start
  constraint horizontal L214
  constraint vertical L215
  constraint horizontal L216
  constraint vertical L217
  constraint coincident L90.end L91.start
  constraint horizontal L218
  constraint vertical L219
  constraint horizontal L220
  constraint vertical L221
  constraint coincident L96.end L97.start
  constraint horizontal L222
  constraint vertical L223
  constraint horizontal L224
  constraint vertical L225
  constraint coincident L95.end L96.start
  constraint horizontal L226
  constraint vertical L227
  constraint horizontal L228
  constraint vertical L229
  constraint coincident L94.start L97.end
  constraint horizontal L230
  constraint vertical L231
  constraint horizontal L232
  constraint vertical L233
  constraint coincident L94.end L95.start
  constraint horizontal L234
  constraint vertical L235
  constraint horizontal L236
  constraint vertical L237
  constraint coincident L88.end L89.start
  constraint horizontal L238
  constraint vertical L239
  constraint horizontal L240
  constraint vertical L241
  constraint coincident L87.end L88.start
  constraint horizontal L242
  constraint vertical L243
  constraint horizontal L244
  constraint vertical L245
  constraint coincident L86.start L89.end
  constraint horizontal L246
  constraint vertical L247
  constraint horizontal L248
  constraint vertical L249
  constraint coincident L86.end L87.start
  constraint horizontal L250
  constraint vertical L251
  constraint horizontal L252
  constraint vertical L253
  constraint coincident L194.end L195.start
  constraint horizontal L254
  constraint vertical L255
  constraint horizontal L256
  constraint vertical L257
  constraint coincident L191.end L192.start
  constraint horizontal L258
  constraint vertical L259
  constraint horizontal L260
  constraint vertical L261
  constraint coincident L182.end L183.start
  constraint horizontal L262
  constraint vertical L263
  constraint horizontal L264
  constraint vertical L265
  constraint coincident L185.end L186.start
  constraint horizontal L266
  constraint vertical L267
  constraint horizontal L268
  constraint vertical L269
  constraint coincident L173.end L174.start
  constraint horizontal L270
  constraint vertical L271
  constraint horizontal L272
  constraint vertical L273
  constraint coincident L176.end L177.start
  constraint horizontal L274
  constraint vertical L275
  constraint horizontal L276
  constraint vertical L277
  constraint coincident L165.end L166.start
  constraint horizontal L278
  constraint vertical L279
  constraint horizontal L280
  constraint vertical L281
  constraint coincident L164.end L165.start
  constraint horizontal L282
  constraint vertical L283
  constraint horizontal L284
  constraint vertical L285
  constraint coincident L166.end L167.start
  constraint horizontal L286
  constraint vertical L287
  constraint horizontal L288
  constraint vertical L289
  constraint coincident L163.end L164.start
  measures "d196" distance of L92.end L198.end
  measures "d197" distance of L92.end L200.end
  measures "d198" distance of L90.start L206.end
  measures "d199" distance of L90.start L208.end
  measures "d200" distance of L91.end L210.end
  measures "d201" distance of L91.end L212.end
  measures "d202" distance of L90.end L214.end
  measures "d203" distance of L90.end L216.end
  measures "d204" distance of L96.end L218.end
  measures "d205" distance of L96.end L220.end
  measures "d206" distance of L95.end L222.end
  measures "d207" distance of L95.end L224.end
  measures "d208" distance of L94.start L226.end
  measures "d209" distance of L94.start L228.end
  measures "d210" distance of L94.end L230.end
  measures "d211" distance of L94.end L232.end
  measures "d212" distance of L88.end L234.end
  measures "d213" distance of L88.end L236.end
  measures "d214" distance of L87.end L238.end
  measures "d215" distance of L87.end L240.end
  measures "d216" distance of L86.start L242.end
  measures "d217" distance of L86.start L244.end
  measures "d218" distance of L86.end L246.end
  measures "d219" distance of L86.end L248.end
  measures "d220" distance of L194.end L250.end
  measures "d221" distance of L194.end L252.end
  measures "d222" distance of L191.end L254.end
  measures "d223" distance of L191.end L256.end
  measures "d224" distance of L182.end L258.end
  measures "d225" distance of L182.end L260.end
  measures "d226" distance of L185.end L262.end
  measures "d227" distance of L185.end L264.end
  measures "d228" distance of L173.end L266.end
  measures "d229" distance of L173.end L268.end
  measures "d230" distance of L176.end L270.end
  measures "d231" distance of L176.end L272.end
  measures "d232" distance of L165.end L274.end
  measures "d233" distance of L165.end L276.end
  measures "d234" distance of L164.end L278.end
  measures "d235" distance of L164.end L280.end
  measures "d236" distance of L166.end L282.end
  measures "d237" distance of L166.end L284.end
  measures "d238" distance of L163.end L286.end
  measures "d239" distance of L163.end L288.end
  measures "d240" diameter of A4
  measures "d243" diameter of A5
  measures "d244" diameter of A6
  measures "d245" diameter of A7
  measures "d246" diameter of A8
  measures "d247" diameter of A9
  measures "d248" diameter of A10
  measures "d249" diameter of A11
  measures "d250" diameter of A12
  measures "d251" diameter of A13
  measures "d252" diameter of A14
  measures "d253" diameter of A15
  measures "d254" diameter of A16
  measures "d255" diameter of A17
  measures "d256" diameter of A18
  measures "d257" diameter of A19
  measures "d258" diameter of A20
  measures "d259" diameter of A21
  measures "d260" diameter of A22
  measures "d261" diameter of A23
  measures "d262" diameter of A24
  measures "d263" diameter of A25
extrude "Extruir15" add sketch "Boceto15" along normal blind 2.5 contours L86 L89 L242 L243 L244 L245 | L86 L87 L246 L247 L248 L249 | L88 L89 L234 L235 L236 L237 | L87 L88 L238 L239 L240 L241 | L90 L93 L203 L204 L206 L207 L208 L209 | L90 L91 L202 L203 L214 L215 L216 L217 | L92 L93 L198 L199 L200 L201 L204 L205 | L91 L92 L202 L205 L210 L211 L212 L213 | L94 L97 L226 L227 L228 L229 | L94 L95 L230 L231 L232 L233 | L96 L97 L218 L219 L220 L221 | L95 L96 L222 L223 L224 L225 | L163 L164 L286 L287 L288 L289 | L194 L195 L250 L251 L252 L253 | L164 L165 L278 L279 L280 L281 | L165 L166 L274 L275 L276 L277 | L191 L192 L254 L255 L256 L257 | L166 L167 L282 L283 L284 L285 | L185 L186 L262 L263 L264 L265 | L173 L174 L266 L267 L268 L269 | L182 L183 L258 L259 L260 L261 | L176 L177 L270 L271 L272 L273
extrude "Extruir16" add 1 faces at (106.6667, 26.6667, 0) along direction (0, 0, -1) blind 2
equation "d193 = Text1-Text"
equation "d268 = ( 1.5 / 2 ) * 1 mm"
